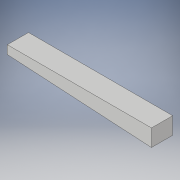
# Autodesk Inventor part: FoldLiftPart1
Saved by Autodesk Inventor 2017 (Build 210142000, 142)
## iProperties
Created: 2017-11-15
Part Number: FoldLiftPart1
Material: Generic
Document SubType Name: Modeling
Designer: User
Density: 1 g/cm^3
Appearance: Default
Author: User
Autodesk Inventor part; units mm, degrees
ref_plane "YZ Plane" through (0, 0, 0) normal (1, 0, 0) x (0, 1, 0)
ref_plane "XZ Plane" through (0, 0, 0) normal (0, 1, 0) x (-1, 0, 0)
ref_plane "XY Plane" through (0, 0, 0) normal (0, 0, 1) x (1, 0, 0)
sketch "Sketch1" plane through (0, 0, 0) normal (0, 0, 1) x (1, 0, 0)
  line L0 (0, 0) -> (-431.8, 0)
  line L1 (0, 0) -> (0, -50.8)
  line L2 (-431.8, 0) -> (-431.8, -25.4)
  line L3 (0, -50.8) -> (-431.8, -25.4)
  line L4 (0, -25.4) -> (-50.8, -25.4)
  line L5 (-50.8, -25.4) -> (-50.8, -12.7)
  line L6 (-50.8, -12.7) -> (0, -12.7)
  line L7 (0, -25.4) -> (0, -12.7)
  dimension "d0" = 431.8
  dimension "d1" = 50.8
  dimension "d4" = 25.4
  dimension "d5" = 50.8
  constraints: 16 end point, 2 perpendicular, 2 vertical, 1 collinear, 1 horizontal, 1 midpoint, 1 point on line
  measures "d0" distance of L0.start L0.end
  measures "d1" distance of L0.start L1.end
  measures "d4" distance of L0.end L2.end
  measures "d5" distance of L4.start L4.end
extrude "Extrusion1" add sketch "Sketch1" along normal blind 63.5
body "Solid1"
